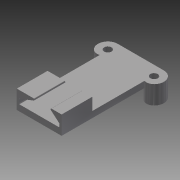
# Autodesk Inventor part: Bluetooth Mount (Improved)
Saved by Autodesk Inventor 2015 (Build 190159000, 159)
## iProperties
Created: 2014-11-14
Part Number: Bluetooth Mount (Improved)
Material: Steel, Mild
Document SubType Name: Modeling
Designer: PLTW
Density: 7.85 g/cm^3
Appearance: Semi-Polished
Author: PLTW
Autodesk Inventor part; units mm, degrees
ref_plane "YZ Plane" through (0, 0, 0) normal (1, 0, 0) x (0, 1, 0)
ref_plane "XZ Plane" through (0, 0, 0) normal (0, 1, 0) x (-1, 0, 0)
ref_plane "XY Plane" through (0, 0, 0) normal (0, 0, 1) x (1, 0, 0)
sketch "Sketch1" plane through (0, 0, 0) normal (0, 1, 0) x (-1, 0, 0)
  line L0 (0, 0) -> (18.4912, 0)
  line L1 (18.7706, -41.900384) -> (-0.2794, -41.900384)
  circle A0 centre (18.7706, -37.836384) radius 1.524
  circle A1 centre (-0.2794, -37.836384) radius 1.524
  arc A2 (18.7706, -41.900384) -> (18.4912, -33.782) centre (18.7706, -37.836384) ccw
  arc A3 (0, -33.782) -> (-0.2794, -41.900384) centre (-0.2794, -37.836384) ccw
  line L2 (18.4912, 0) -> (18.4912, -33.782)
  line L3 (0, -33.782) -> (0, 0)
  dimension "d0" = 18.4912
  dimension "d2" = 3.048
  dimension "d12" = 33.782
  dimension "d13" = 19.05
  dimension "d14" = 2.54
  constraints: 8 end point, 4 centre point, 4 point on circle, 2 concentric, 2 equal radius, 2 horizontal alignment, 2 parallel, 1 horizontal, 1 perpendicular, 1 tangent
  measures "d0" distance of L0.start L0.end
  measures "d2" diameter of A0
  measures "d12" distance of L0.end L2.end
  measures "d13" distance of A1.centre A0.centre
  measures "d14" radial gap between concentric circles of A2 A0
extrude "Extrusion1" add sketch "Sketch1" along normal blind 2.54
sketch "Sketch3" plane through (0, 2.54, 0) normal (0, 1, 0) x (1, 0, 0)
  line L0 (-18.4912, 33.782) -> (-18.4912, 0) projected
  line L1 (0, 0) -> (0, 33.782) projected
  line L2 (-18.4912, 0) -> (0, 0) projected
  line L3 (-1.27, -2.54) -> (-1.27, 33.02) projected
  line L4 (-17.2212, 33.02) -> (-17.2212, -2.54) projected
  line L5 (-18.4912, 0) -> (-17.6022, 0)
  line L6 (-17.6022, 0) -> (-17.6022, 12.7)
  line L7 (-17.6022, 12.7) -> (-18.4912, 12.7)
  line L8 (-18.4912, 12.7) -> (-18.4912, 0)
  line L9 (0, 0) -> (-0.889, 0)
  line L10 (-0.889, 0) -> (-0.889, 12.7)
  line L11 (-0.889, 12.7) -> (0, 12.7)
  line L12 (0, 12.7) -> (0, 0)
  dimension "d15" = 0.381
  dimension "d16" = 12.7
  constraints: 16 end point, 4 parallel, 2 equal length, 2 horizontal, 2 perpendicular
  measures "d15" distance between parallel lines of L10 L3
  measures "d16" distance between parallel lines of L2 L11
extrude "Extrusion2" add sketch "Sketch3" along normal blind 5.08
fillet "Fillet1" radius 0.381 2 edges at (-0.889, 2.54, -6.35) (-17.6022, 2.54, -6.35)
sketch "Sketch4" plane through (0, 7.62, -12.7) normal (0, 0, -1) x (-1, 0, 0)
  line L0 (1.27, -5.08) -> (0, -5.08)
  arc A0 (0.889, -4.699) -> (1.27, -5.08) centre (1.27, -4.699) ccw
  line L1 (0.889, -4.699) -> (0.889, 0)
  line L2 (0, 0) -> (0.889, 0)
  line L3 (0, -5.08) -> (0, 0)
  line L4 (18.4912, -5.08) -> (17.2212, -5.08)
  line L5 (18.4912, -5.08) -> (18.4912, 0)
  line L6 (17.6022, 0) -> (18.4912, 0)
  line L7 (17.6022, -4.699) -> (17.6022, 0)
  arc A1 (17.2212, -5.08) -> (17.6022, -4.699) centre (17.2212, -4.699) ccw
  line L8 (15.6591, -3.683) -> (2.8321, -3.683)
  line L9 (15.6591, -3.683) -> (15.6591, -2.667)
  line L10 (2.8321, -2.667) -> (15.6591, -2.667)
  line L11 (2.8321, -3.683) -> (2.8321, -2.667)
  line L12 (11.8237, -2.667) -> (3.4417, -2.667)
  line L13 (11.8237, -2.667) -> (11.8237, -1.8288)
  line L14 (3.4417, -1.8288) -> (11.8237, -1.8288)
  line L15 (3.4417, -2.667) -> (3.4417, -1.8288)
  line L16 (1.27, -5.08) -> (17.2212, -5.08)
  line L17 (17.2212, -5.08) -> (17.2212, -3.683)
  line L18 (1.27, -3.683) -> (17.2212, -3.683)
  line L19 (1.27, -5.08) -> (1.27, -3.683)
  line L20 (14.3637, -2.667) -> (12.3317, -2.667)
  line L21 (14.3637, -2.667) -> (14.3637, -2.159)
  line L22 (12.3317, -2.159) -> (14.3637, -2.159)
  line L23 (12.3317, -2.667) -> (12.3317, -2.159)
  line L24 (13.1953, -2.667) -> (12.8143, -2.667)
  line L25 (13.1953, -2.667) -> (13.1953, -1.905)
  line L26 (12.8143, -1.905) -> (13.1953, -1.905)
  line L27 (12.8143, -2.667) -> (12.8143, -1.905)
  line L28 (0.889, 0) -> (5.192475, 0)
  line L29 (17.6022, -4.699) -> (17.6022, 0)
  line L30 (0.889, -4.699) -> (0.889, 0)
  line L31 (0.889, -3.674312) -> (5.192475, 0)
  line L32 (17.6022, 0) -> (9.553974, 0)
  line L33 (9.553974, 0) -> (17.6022, -3.156167)
  point P0 (0, -7.62)
extrude "Extrusion3" add sketch "Sketch4" against normal up to surface (12.7 mm away) contours L1 L28 L31 | L33 L32 L7
fillet "Fillet2" radius 0.381 4 edges at (-5.1925, 7.62, -6.35) (-9.554, 7.62, -6.35) (-0.889, 3.9457, -6.35) (-17.6022, 4.4638, -6.35)
sketch "Sketch5" plane through (0, 0, 0) normal (0, -1, 0) x (1, 0, 0)
  circle A0 centre (0.2794, -37.836384) radius 1.524
  circle A1 centre (-18.7706, -37.836384) radius 1.524
  line L0 (0, 0) -> (-18.4912, 0)
  line L1 (-18.4912, 0) -> (-18.4912, -33.782)
  arc A2 (-18.4912, -33.782) -> (-18.7706, -41.900384) centre (-18.7706, -37.836384) ccw
  line L2 (-18.7706, -41.900384) -> (0.2794, -41.900384)
  arc A3 (0.2794, -41.900384) -> (0, -33.782) centre (0.2794, -37.836384) ccw
  line L3 (0, -33.782) -> (0, 0)
  circle A4 centre (0.2794, -37.836384) radius 1.524
  circle A5 centre (0.2794, -37.836384) radius 4.064
  circle A6 centre (-18.7706, -37.836384) radius 1.524
  circle A7 centre (-18.7706, -37.836384) radius 4.064
  constraints: 2 centre point, 2 coincident, 2 concentric
extrude "Extrusion4" add sketch "Sketch5" along normal blind 5.08 contours A3 A5 | A7 A2
sketch "Sketch6" plane through (0, 0, 0) normal (0, -1, 0) x (1, 0, 0)
  arc A0 (0, -33.782) -> (0.2794, -41.900384) centre (0.2794, -37.836384) ccw
  line L0 (0, -33.782) -> (0, 0)
  line L1 (0, 0) -> (-18.4912, 0)
  line L2 (-18.4912, 0) -> (-18.4912, -33.782)
  arc A1 (-18.7706, -41.900384) -> (-18.4912, -33.782) centre (-18.7706, -37.836384) ccw
  line L3 (-18.7706, -41.900384) -> (0.2794, -41.900384)
  line L4 (-2.2606, -18.966015) -> (-16.2306, -18.966015)
  line L5 (-16.2306, -18.966015) -> (-16.2306, -41.900384)
  line L6 (-16.2306, -41.900384) -> (-2.2606, -41.900384)
  line L7 (-2.2606, -41.900384) -> (-2.2606, -18.966015)
  line L8 (-18.7706, -41.900384) -> (0.2794, -41.900384)
  point P0 (-9.2456, -41.900384)
  point P1 (-9.2456, -41.900384)
  dimension "d29" = 13.97
  constraints: 8 end point, 2 midpoint, 2 parallel, 1 coincident, 1 horizontal, 1 perpendicular, 1 point on line
  measures "d29" distance of L4.start L4.end
extrude "Extrusion5" cut sketch "Sketch6" along normal blind 25.4 contours L7 A0 | A0 L7 L3 L5 A1 L4 | A1 L5
fillet "Fillet3" radius 3.175 4 edges at (-2.2606, -2.54, -41.0088) (-2.2606, -2.54, -34.6639) (-16.2306, -2.54, -41.0088) (-16.2306, -2.54, -34.6639)
body "Solid1"
